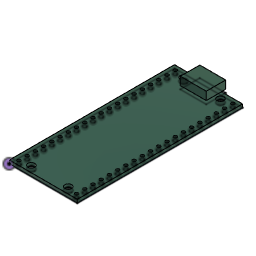
Pi Pico v3 (Autodesk Fusion 360 design; units mm, degrees)
Autodesk Fusion 360 part; units mm, degrees
sketch "Skizze1" plane through (0, 0, 0) normal (0, 0, 1) x (1, 0, 0)
  line L0 (0, 0) -> (21, 0)
  line L1 (21, 0) -> (21, 51)
  line L2 (21, 51) -> (0, 51)
  line L3 (0, 51) -> (0, 0)
  circle A0 centre (4.8, 49) radius 1.05
  circle A1 centre (16.2, 49) radius 1.05
  circle A2 centre (4.8, 2) radius 1.05
  circle A3 centre (16.2, 2) radius 1.05
  line L4 (6.5, 52.3) -> (14.5, 52.3)
  line L5 (14.5, 52.3) -> (14.5, 46.3)
  line L6 (14.5, 46.3) -> (6.5, 46.3)
  line L7 (6.5, 46.3) -> (6.5, 52.3)
  circle A4 centre (1.61, 49.63) radius 0.5
  circle A5 centre (19.39, 49.63) radius 0.5
  circle A6 centre (1.61, 47.09) radius 0.5
  circle A7 centre (19.39, 47.09) radius 0.5
  circle A8 centre (1.61, 44.55) radius 0.5
  circle A9 centre (19.39, 44.55) radius 0.5
  circle A10 centre (1.61, 42.01) radius 0.5
  circle A11 centre (19.39, 42.01) radius 0.5
  circle A12 centre (1.61, 39.47) radius 0.5
  circle A13 centre (19.39, 39.47) radius 0.5
  circle A14 centre (1.61, 36.93) radius 0.5
  circle A15 centre (19.39, 36.93) radius 0.5
  circle A16 centre (1.61, 34.39) radius 0.5
  circle A17 centre (19.39, 34.39) radius 0.5
  circle A18 centre (1.61, 31.85) radius 0.5
  circle A19 centre (19.39, 31.85) radius 0.5
  circle A20 centre (1.61, 29.31) radius 0.5
  circle A21 centre (19.39, 29.31) radius 0.5
  circle A22 centre (1.61, 26.77) radius 0.5
  circle A23 centre (19.39, 26.77) radius 0.5
  circle A24 centre (1.61, 24.23) radius 0.5
  circle A25 centre (19.39, 24.23) radius 0.5
  circle A26 centre (1.61, 21.69) radius 0.5
  circle A27 centre (19.39, 21.69) radius 0.5
  circle A28 centre (1.61, 19.15) radius 0.5
  circle A29 centre (19.39, 19.15) radius 0.5
  circle A30 centre (1.61, 16.61) radius 0.5
  circle A31 centre (19.39, 16.61) radius 0.5
  circle A32 centre (1.61, 14.07) radius 0.5
  circle A33 centre (19.39, 14.07) radius 0.5
  circle A34 centre (1.61, 11.53) radius 0.5
  circle A35 centre (19.39, 11.53) radius 0.5
  circle A36 centre (1.61, 8.99) radius 0.5
  circle A37 centre (19.39, 8.99) radius 0.5
  circle A38 centre (1.61, 6.45) radius 0.5
  circle A39 centre (19.39, 6.45) radius 0.5
  circle A40 centre (1.61, 3.91) radius 0.5
  circle A41 centre (19.39, 3.91) radius 0.5
  circle A42 centre (1.61, 1.37) radius 0.5
  circle A43 centre (19.39, 1.37) radius 0.5
  dimension "d1" = 21
  dimension "d2" = 51
  dimension "d3" = 2.1
  dimension "d4" = 4.8
  dimension "d5" = 2
  dimension "d8" = 11.4
  dimension "d9" = -47
  dimension "d10" = 8
  dimension "d11" = 6
  dimension "d12" = 1.3
  dimension "d13" = 6.5
  dimension "d20" = 1
  dimension "d21" = 1.37
  dimension "d22" = 1.61
  dimension "d25" = 17.78
  dimension "d26" = -2.54
  constraint horizontal L0
  constraint vertical L1
  constraint horizontal L2
  constraint vertical L3
  constraint coincident L0.start L3.end
  constraint horizontal L4
  constraint vertical L5
  constraint horizontal L6
  constraint vertical L7
  measures "d1" distance of L0.start L0.end
  measures "d2" distance of L0.start L2.end
  measures "d3" diameter of A0
  measures "d4" distance of L3 A0.centre
  measures "d5" distance of L2 A0.centre
  measures "d10" distance of L4.start L4.end
  measures "d11" distance of L4.start L6.end
  measures "d12" distance of L2 L4
  measures "d13" distance of L1 L5
  measures "d20" diameter of A4
  measures "d21" distance of L2 A4.centre
  measures "d22" distance of L3 A4.centre
extrude "Extrusion4" add sketch "Skizze1" along normal blind 1 contours L0 L1 L2 L3 L5 L6 L7
extrude "Extrusion2" add sketch "Skizze1" along normal blind 3.5 contours L2 L4 L5 L7 | L2 L5 L6 L7
extrude "Extrusion3" cut sketch "Skizze1" along normal blind 1 contours L2 L4 L5 L7
